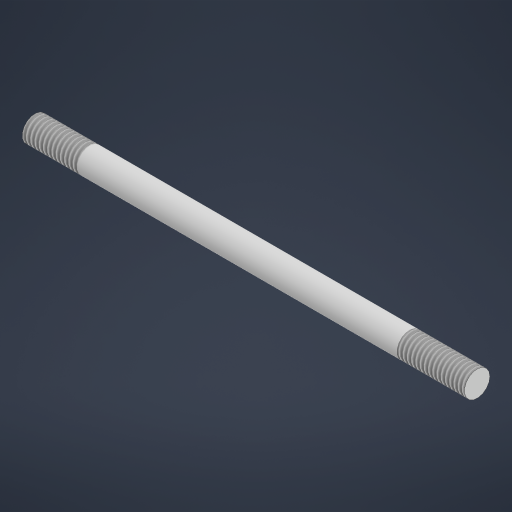
# Autodesk Inventor part: sf_Piston_Rod_1
Saved by Autodesk Inventor 2024 (Build 280153000, 153)
## iProperties
Created: 2024-03-22
Part Number: sf_Piston_Rod_1
Material: Generisch
Document SubType Name: Modeling
Designer: Simon
Density: 1 g/cm^3
Appearance: Vorgabe
Author: Simon
Autodesk Inventor part; units mm, degrees
ref_plane "YZ Plane" through (0, 0, 0) normal (1, 0, 0) x (0, 1, 0)
ref_plane "XZ Plane" through (0, 0, 0) normal (0, 1, 0) x (-1, 0, 0)
ref_plane "XY Plane" through (0, 0, 0) normal (0, 0, 1) x (1, 0, 0)
sketch "Skizze1" plane through (0, 0, 0) normal (1, 0, 0) x (0, 1, 0)
  circle A0 centre (0, 0) radius 3
  dimension "d0" = 6
  constraints: 1 centre point, 1 coincident
  measures "d0" diameter of A0
extrude "Extrusion1" add sketch "Skizze1" along normal mid plane 104.5
thread "Gewinde1" size "M6x1" class "6g" standard "ISO Metric profile" length 13
thread "Gewinde2" size "M6x1" class "6g" standard "ANSI Metric M Profile" length 16
